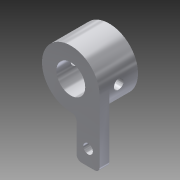
# Autodesk Inventor part: HW 4 Part 6
Saved by Autodesk Inventor 2015 (Build 190159000, 159)
## iProperties
Created: 2016-02-01
Part Number: HW 4 Part 6
Material: Aluminum 6061
Document SubType Name: Modeling
Designer: Melissa
Density: 2.7 g/cm^3
Appearance: Aluminum - Flat
Mass: 64.3881 g
Surface Area: 78.6484 cm^2
Volume: 23.8474 cm^3
Author: Melissa
Autodesk Inventor part; units mm, degrees
ref_plane "YZ Plane" through (0, 0, 0) normal (1, 0, 0) x (0, 1, 0)
ref_plane "XZ Plane" through (0, 0, 0) normal (0, 1, 0) x (-1, 0, 0)
ref_plane "XY Plane" through (0, 0, 0) normal (0, 0, 1) x (1, 0, 0)
sketch "Sketch1" plane through (0, 0, 0) normal (0, 0, 1) x (1, 0, 0)
  arc A0 (19.05, 0) -> (0.5443, -19.0422) centre (0, 0) ccw
  circle A1 centre (0, 0) radius 9.525
  line L0 (19.05, 0) -> (19.05, -41.275)
  line L1 (15.875, -44.45) -> (6.985, -44.45)
  line L2 (3.81, -41.275) -> (3.81, -22.2159)
  circle A2 centre (11.43, -34.29) radius 3.175
  arc A3 (3.81, -41.275) -> (6.985, -44.45) centre (6.985, -41.275) ccw
  arc A4 (15.875, -44.45) -> (19.05, -41.275) centre (15.875, -41.275) ccw
  arc A5 (3.81, -22.2159) -> (0.5443, -19.0422) centre (0.635, -22.2159) ccw
  point P0 (19.05, -44.45)
  point P1 (3.81, -44.45)
  point P2 (3.81, -18.6651)
  dimension "d0" = 38.1
  dimension "d1" = 19.05
  dimension "d2" = 44.45
  dimension "d3" = 15.24
  dimension "d4" = 6.35
  dimension "d5" = 7.62
  dimension "d6" = 10.16
  dimension "d7" = 3.175
  dimension "d8" = 3.175
  constraints: 9 point on circle, 6 centre point, 6 end point, 6 tangent, 5 point on line, 2 coincident, 2 vertical, 1 equal radius, 1 perpendicular
  measures "d0" diameter of A0
  measures "d1" diameter of A1
  measures "d2" distance of L0.start point (19.05, -44.45)
  measures "d3" distance of point (19.05, -44.45) point (3.81, -44.45)
  measures "d4" diameter of A2
  measures "d5" distance from line of L0 A2.centre
  measures "d6" distance from line of L1 A2.centre
  measures "d7" radius of A3
  measures "d8" radius of A5
extrude "Extrusion1" add sketch "Sketch1" along normal blind 6.35
sketch "Sketch2" plane through (0, 0, 0) normal (0, 0, -1) x (-1, 0, 0)
  circle A0 centre (0, 0) radius 19.05
  dimension "d11" = 38.1
  constraints: 1 centre point, 1 coincident
  measures "d11" diameter of A0
extrude "Extrusion2" add sketch "Sketch2" along normal blind 19.05
sketch "Sketch3" plane through (0, 0, -19.05) normal (0, 0, -1) x (-1, 0, 0)
  circle A0 centre (0, 0) radius 9.525
  dimension "d14" = 19.05
  constraints: 1 centre point, 1 coincident
  measures "d14" diameter of A0
extrude "Extrusion3" cut sketch "Sketch3" against normal through all
sketch "Sketch4" plane through (19.05, -41.275, 0) normal (1, 0, 0) x (0, 0, -1)
  circle A0 centre (6.35, 41.275) radius 3.175
  line L0 (19.05, 22.225) -> (19.05, 60.325) projected
  point P0 (0, 41.275)
  dimension "d17" = 6.35
  dimension "d18" = 0
  dimension "d19" = 12.7
  constraints: 1 centre point
  measures "d17" diameter of A0
  measures "d18" vertical distance of point (0, 41.275) A0.centre
  measures "d19" distance from line of L0 A0.centre
extrude "Extrusion4" cut sketch "Sketch4" against normal through all
body "Solid1"
